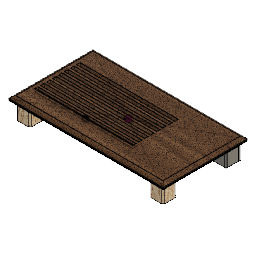
laotop-stand (Autodesk Fusion 360 design; units mm, degrees)
Autodesk Fusion 360 part; units mm, degrees
sketch "Sketch1" plane through (0, 0, 0) normal (0, 0, 1) x (1, 0, 0) in component "Top"
  line L0 (279.4, 152.4) -> (-279.4, 152.4)
  line L1 (-279.4, 152.4) -> (-279.4, -152.4)
  line L2 (-279.4, -152.4) -> (279.4, -152.4)
  line L3 (279.4, -152.4) -> (279.4, 152.4)
  line L4 (279.4, 152.4) -> (-279.4, -152.4) construction
  line L5 (-279.4, 152.4) -> (279.4, -152.4) construction
  line L6 (101.6, -84.6667) -> (-254, -84.6667)
  line L7 (-254, -84.6667) -> (-254, -71.9667)
  line L8 (-254, -71.9667) -> (101.6, -71.9667)
  line L9 (101.6, -71.9667) -> (101.6, -84.6667)
  line L10 (101.6, -84.6667) -> (-254, -71.9667) construction
  line L11 (-254, -84.6667) -> (101.6, -71.9667) construction
  point P0 (-76.2, -78.3167)
  dimension "d17" = 558.8
  dimension "d18" = 304.8
  dimension "d19" = 67.7333
  dimension "d20" = 25.4
  dimension "d21" = 355.6
  dimension "d22" = 12.7
  constraint perpendicular L0 L1
  constraint parallel L0 L2
  constraint parallel L1 L3
  constraint horizontal L0
  constraint coincident L4 origin
  constraint coincident L5 origin
  constraint perpendicular L6 L7
  constraint parallel L6 L8
  constraint parallel L7 L9
  constraint horizontal L6
  constraint coincident L10 P0
  constraint coincident L11 P0
  measures "d17" distance of L1.end L2.end
  measures "d18" distance of L0.end L1.end
  measures "d19" distance of L2 L6
  measures "d20" distance of L1 L7
  measures "d21" distance of L6.start L6.end
  measures "d22" distance of L6.end L7.end
extrude "Extrude1" add sketch "Sketch1" along normal mid plane 19.05 makes body 1 in component "Top"
pattern_linear "R-Pattern1" count 1 spacing 0 along (1, 0, 0) count 8 spacing 21.7714 along (0, 1, 0) of 4 faces at (-16.9333, -71.9667, -3.175) (-135.4667, -84.6667, -3.175) (-254, -80.4333, -3.175) (101.6, -76.2, -3.175) on bodies 1 in component "Top"
sketch "Sketch1 (2)" plane through (0, 0, -9.525) normal (0, 0, -1) x (-1, 0, 0) in component "Leg 1"
  line L0 (254, -67.7333) -> (254, -80.4333)
  line L1 (254, -80.4333) -> (-101.6, -80.4333)
  line L2 (-101.6, -80.4333) -> (-101.6, -67.7333)
  line L3 (-101.6, -67.7333) -> (254, -67.7333)
  line L4 (254, -45.9619) -> (254, -58.6619)
  line L5 (254, -58.6619) -> (-101.6, -58.6619)
  line L6 (-101.6, -58.6619) -> (-101.6, -45.9619)
  line L7 (-101.6, -45.9619) -> (254, -45.9619)
  line L8 (254, -24.1905) -> (254, -36.8905)
  line L9 (254, -36.8905) -> (-101.6, -36.8905)
  line L10 (-101.6, -36.8905) -> (-101.6, -24.1905)
  line L11 (-101.6, -24.1905) -> (254, -24.1905)
  line L12 (254, -2.419) -> (254, -15.119)
  line L13 (254, -15.119) -> (-101.6, -15.119)
  line L14 (-101.6, -15.119) -> (-101.6, -2.419)
  line L15 (-101.6, -2.419) -> (254, -2.419)
  line L16 (254, 19.3524) -> (254, 6.6524)
  line L17 (254, 6.6524) -> (-101.6, 6.6524)
  line L18 (-101.6, 6.6524) -> (-101.6, 19.3524)
  line L19 (-101.6, 19.3524) -> (254, 19.3524)
  line L20 (254, 41.1238) -> (254, 28.4238)
  line L21 (254, 28.4238) -> (-101.6, 28.4238)
  line L22 (-101.6, 28.4238) -> (-101.6, 41.1238)
  line L23 (-101.6, 41.1238) -> (254, 41.1238)
  line L24 (254, 62.8952) -> (254, 50.1952)
  line L25 (254, 50.1952) -> (-101.6, 50.1952)
  line L26 (-101.6, 50.1952) -> (-101.6, 62.8952)
  line L27 (-101.6, 62.8952) -> (254, 62.8952)
  line L28 (254, 71.9667) -> (-101.6, 71.9667)
  line L29 (-101.6, 71.9667) -> (-101.6, 84.6667)
  line L30 (-101.6, 84.6667) -> (254, 84.6667)
  line L31 (254, 84.6667) -> (254, 71.9667)
  line L32 (-279.4, 152.4) -> (-279.4, -152.4)
  line L33 (-279.4, -152.4) -> (279.4, -152.4)
  line L34 (279.4, -152.4) -> (279.4, 152.4)
  line L35 (279.4, 152.4) -> (-279.4, 152.4)
  line L36 (-215.9, -139.7) -> (-266.7, -139.7)
  line L37 (-266.7, -139.7) -> (-266.7, -88.9)
  line L38 (-266.7, -88.9) -> (-215.9, -88.9)
  line L39 (-215.9, -88.9) -> (-215.9, -139.7)
  line L40 (-279.4, 152.4) -> (-279.4, -152.4)
  line L41 (-279.4, -152.4) -> (279.4, -152.4)
  line L42 (-222.25, -131.2333) -> (-260.35, -131.2333)
  line L43 (-260.35, -131.2333) -> (-260.35, -121.0733)
  line L44 (-260.35, -121.0733) -> (-222.25, -121.0733)
  line L45 (-222.25, -121.0733) -> (-222.25, -131.2333)
  line L46 (-279.4, 152.4) -> (-279.4, -152.4)
  line L47 (-266.7, -114.3) -> (-215.9, -114.3) construction
  line L48 (-260.35, -107.5267) -> (-222.25, -107.5267)
  line L49 (-260.35, -97.3667) -> (-260.35, -107.5267)
  line L50 (-222.25, -97.3667) -> (-260.35, -97.3667)
  line L51 (-222.25, -107.5267) -> (-222.25, -97.3667)
  line L52 (-279.4, 0) -> (279.4, 0) construction
  line L53 (-266.7, 88.9) -> (-215.9, 88.9)
  line L54 (-222.25, 97.3667) -> (-260.35, 97.3667)
  line L55 (-266.7, 114.3) -> (-215.9, 114.3) construction
  line L56 (-222.25, 131.2333) -> (-260.35, 131.2333)
  line L57 (-215.9, 139.7) -> (-266.7, 139.7)
  line L58 (-215.9, 88.9) -> (-215.9, 139.7)
  line L59 (-222.25, 121.0733) -> (-222.25, 131.2333)
  line L60 (-260.35, 97.3667) -> (-260.35, 107.5267)
  line L61 (-222.25, 107.5267) -> (-222.25, 97.3667)
  line L62 (-260.35, 121.0733) -> (-222.25, 121.0733)
  line L63 (-260.35, 107.5267) -> (-222.25, 107.5267)
  line L64 (-260.35, 131.2333) -> (-260.35, 121.0733)
  line L65 (-266.7, 139.7) -> (-266.7, 88.9)
  line L66 (0, -152.4) -> (0, 152.4) construction
  line L67 (266.7, -139.7) -> (266.7, -88.9)
  line L68 (222.25, -121.0733) -> (222.25, -131.2333)
  line L69 (222.25, -107.5267) -> (222.25, -97.3667)
  line L70 (222.25, -131.2333) -> (260.35, -131.2333)
  line L71 (222.25, -97.3667) -> (260.35, -97.3667)
  line L72 (266.7, -88.9) -> (215.9, -88.9)
  line L73 (260.35, -107.5267) -> (222.25, -107.5267)
  line L74 (215.9, -139.7) -> (266.7, -139.7)
  line L75 (260.35, -121.0733) -> (222.25, -121.0733)
  line L76 (260.35, -131.2333) -> (260.35, -121.0733)
  line L77 (260.35, -97.3667) -> (260.35, -107.5267)
  line L78 (215.9, -88.9) -> (215.9, -139.7)
  line L79 (266.7, -114.3) -> (215.9, -114.3) construction
  line L80 (260.35, 107.5267) -> (222.25, 107.5267)
  line L81 (222.25, 131.2333) -> (260.35, 131.2333)
  line L82 (260.35, 131.2333) -> (260.35, 121.0733)
  line L83 (222.25, 121.0733) -> (222.25, 131.2333)
  line L84 (260.35, 97.3667) -> (260.35, 107.5267)
  line L85 (222.25, 97.3667) -> (260.35, 97.3667)
  line L86 (266.7, 139.7) -> (266.7, 88.9)
  line L87 (215.9, 139.7) -> (266.7, 139.7)
  line L88 (215.9, 88.9) -> (215.9, 139.7)
  line L89 (260.35, 121.0733) -> (222.25, 121.0733)
  line L90 (266.7, 88.9) -> (215.9, 88.9)
  line L91 (222.25, 107.5267) -> (222.25, 97.3667)
  line L92 (266.7, 114.3) -> (215.9, 114.3) construction
  line L93 (254, 80.4333) -> (254, 67.7333)
  line L94 (254, 67.7333) -> (-101.6, 67.7333)
  line L95 (-101.6, 67.7333) -> (-101.6, 80.4333)
  line L96 (-101.6, 80.4333) -> (254, 80.4333)
  line L97 (254, 58.6619) -> (254, 45.9619)
  line L98 (254, 45.9619) -> (-101.6, 45.9619)
  line L99 (-101.6, 45.9619) -> (-101.6, 58.6619)
  line L100 (-101.6, 58.6619) -> (254, 58.6619)
  line L101 (254, 36.8905) -> (254, 24.1905)
  line L102 (254, 24.1905) -> (-101.6, 24.1905)
  line L103 (-101.6, 24.1905) -> (-101.6, 36.8905)
  line L104 (-101.6, 36.8905) -> (254, 36.8905)
  line L105 (254, 15.119) -> (254, 2.419)
  line L106 (254, 2.419) -> (-101.6, 2.419)
  line L107 (-101.6, 2.419) -> (-101.6, 15.119)
  line L108 (-101.6, 15.119) -> (254, 15.119)
  line L109 (254, -6.6524) -> (254, -19.3524)
  line L110 (254, -19.3524) -> (-101.6, -19.3524)
  line L111 (-101.6, -19.3524) -> (-101.6, -6.6524)
  line L112 (-101.6, -6.6524) -> (254, -6.6524)
  line L113 (254, -28.4238) -> (254, -41.1238)
  line L114 (254, -41.1238) -> (-101.6, -41.1238)
  line L115 (-101.6, -41.1238) -> (-101.6, -28.4238)
  line L116 (-101.6, -28.4238) -> (254, -28.4238)
  line L117 (254, -50.1952) -> (254, -62.8952)
  line L118 (254, -62.8952) -> (-101.6, -62.8952)
  line L119 (-101.6, -62.8952) -> (-101.6, -50.1952)
  line L120 (-101.6, -50.1952) -> (254, -50.1952)
  line L121 (-101.6, -71.9667) -> (254, -71.9667)
  line L122 (254, -71.9667) -> (254, -84.6667)
  line L123 (254, -84.6667) -> (-101.6, -84.6667)
  line L124 (-101.6, -84.6667) -> (-101.6, -71.9667)
  line L125 (-279.4, 152.4) -> (-279.4, -152.4)
  line L126 (-279.4, -152.4) -> (279.4, -152.4)
  line L127 (279.4, -152.4) -> (279.4, 152.4)
  line L128 (279.4, 152.4) -> (-279.4, 152.4)
  dimension "d31" = 50.8
  dimension "d32" = 50.8
  dimension "d33" = 12.7
  dimension "d34" = 12.7
  dimension "d36" = 10.16
  dimension "d39" = 8.4667
  dimension "d40" = 6.35
  dimension "d41" = 6.35
  constraint horizontal L36
  constraint vertical L37
  constraint horizontal L38
  constraint vertical L39
  constraint horizontal L42
  constraint vertical L43
  constraint horizontal L44
  constraint vertical L45
  constraint midpoint L37 L47.start
  constraint midpoint L39 L47.end
  constraint symmetric L42.start L47 L50.start
  constraint symmetric L42.end L47 L49.start
  constraint symmetric L43.end L47 L48.start
  constraint symmetric L44.end L47 L48.end
  constraint midpoint L32 L52.start
  constraint midpoint L34 L52.end
  constraint symmetric L36.start L52 L57.start
  constraint symmetric L36.end L52 L57.end
  constraint symmetric L37.end L52 L53.start
  constraint symmetric L38.end L52 L53.end
  constraint symmetric L42.start L52 L56.start
  constraint symmetric L42.end L52 L56.end
  constraint symmetric L43.end L52 L62.start
  constraint symmetric L44.end L52 L59.start
  constraint symmetric L47.start L52 L55.start
  constraint symmetric L47.end L52 L55.end
  constraint symmetric L48.start L52 L60.end
  constraint symmetric L48.end L52 L61.start
  constraint symmetric L49.start L52 L54.end
  constraint symmetric L50.start L52 L54.start
  constraint midpoint L41 L66.start
  constraint midpoint L35 L66.end
  constraint symmetric L36.start L66 L74.start
  constraint symmetric L36.end L66 L67.start
  constraint symmetric L37.end L66 L67.end
  constraint symmetric L38.end L66 L72.end
  constraint symmetric L42.start L66 L68.end
  constraint symmetric L42.end L66 L70.end
  constraint symmetric L43.end L66 L75.start
  constraint symmetric L44.end L66 L68.start
  constraint symmetric L47.start L66 L79.start
  constraint symmetric L47.end L66 L79.end
  constraint symmetric L48.start L66 L73.start
  constraint symmetric L48.end L66 L69.start
  constraint symmetric L49.start L66 L71.end
  constraint symmetric L50.start L66 L69.end
  constraint symmetric L62.start L66 L82.end
  constraint symmetric L57.end L66 L86.start
  constraint symmetric L53.start L66 L86.end
  constraint symmetric L56.end L66 L81.end
  constraint symmetric L56.start L66 L81.start
  constraint symmetric L53.end L66 L88.start
  constraint symmetric L54.start L66 L85.start
  constraint symmetric L54.end L66 L84.start
  constraint symmetric L61.start L66 L80.end
  constraint symmetric L60.end L66 L80.start
  constraint symmetric L55.end L66 L92.end
  constraint symmetric L55.start L66 L92.start
  constraint symmetric L57.start L66 L87.start
  constraint symmetric L59.start L66 L83.start
  measures "d31" distance of L36.start L36.end
  measures "d32" distance of L36.start L38.end
  measures "d33" distance of L37 L40
  measures "d34" distance of L36 L41
  measures "d36" distance of L42.start L44.end
  measures "d39" distance of L36 L42
  measures "d40" distance of L37 L43
  measures "d41" distance of L39 L45
extrude "Extrude1'" add sketch "Sketch1 (2)" along normal blind 57.15 separate body contours L53 L57 L58 L65 | L54 L60 L61 L63 | L56 L59 L62 L64 makes body 2 in component "Leg 1"
extrude "Extrude2" add sketch "Sketch1 (2)" against normal blind 12.7 separate body contours L54 L60 L61 L63 | L56 L59 L62 L64 makes body 3 at (247.65, 121.0733, -5.2917) makes body 4 at (234.95, 97.3667, -5.2917) in component "Leg 1"
combine "Combine1" operation add target body 3 tool bodies 4 2 keep tools in component "Leg 1"
combine "Combine2" operation add target body 4 tool bodies 2 3 keep tools in component "Leg 1"
combine "Combine1'" operation add target body 1 tool bodies 3 keep tools in component "Top"
combine "Combine2'" operation cut target body 1 tool bodies 4 keep tools in component "Top"
extrude "Extrude3" add sketch "Sketch1 (2)" along normal blind 57.15 separate body contours L36 L37 L38 L39 | L42 L43 L44 L45 | L48 L49 L50 L51 makes body 5 in component "Leg 1"
extrude "Extrude4" add sketch "Sketch1 (2)" against normal blind 12.7 contours L42 L43 L44 L45 | L48 L49 L50 L51 bodies 5 in component "Leg 1"
combine "Combine3" operation cut target body 1 tool bodies 5 keep tools in component "Top"
extrude "Extrude5" add sketch "Sketch1 (2)" along normal blind 57.15 separate body contours L67 L72 L74 L78 | L68 L70 L75 L76 | L69 L71 L73 L77 makes body 6 in component "Leg 1"
extrude "Extrude6" add sketch "Sketch1 (2)" against normal blind 12.7 contours L68 L70 L75 L76 | L69 L71 L73 L77 bodies 6 in component "Leg 1"
combine "Combine4" operation cut target body 1 tool bodies 6 keep tools in component "Top"
extrude "Extrude7" add sketch "Sketch1 (2)" along normal blind 57.15 separate body contours L80 L84 L85 L91 | L81 L82 L83 L89 | L86 L87 L88 L90 makes body 7 in component "Leg 1"
extrude "Extrude8" add sketch "Sketch1 (2)" against normal blind 12.7 contours L80 L84 L85 L91 | L81 L82 L83 L89 bodies 7 in component "Leg 1"
combine "Combine5" operation cut target body 1 tool bodies 7 keep tools in component "Top"
fillet "Fillet1" radius 12.7 4 edges at (0, 152.4, 9.525) (-279.4, 0, 9.525) (0, -152.4, 9.525) (279.4, 0, 9.525) on bodies 1 in component "Top"
chamfer "Chamfer1" distance 6.35 angle 45 16 edges at (266.7, 139.7, -38.1) (266.7, 88.9, -38.1) (215.9, 139.7, -38.1) (215.9, 88.9, -38.1) (-215.9, -139.7, -38.1) (-215.9, -88.9, -38.1) (-266.7, -139.7, -38.1) (-266.7, -88.9, -38.1) (215.9, -88.9, -38.1) (215.9, -139.7, -38.1) (266.7, -139.7, -38.1) (266.7, -88.9, -38.1) (-215.9, 88.9, -38.1) (-215.9, 139.7, -38.1) (-266.7, 88.9, -38.1) (-266.7, 139.7, -38.1) on bodies 4 5 6 7 in component "Leg 1"
chamfer "Chamfer1'" distance 3.175 angle 45 4 edges at (279.4, 0, -9.525) (0, -152.4, -9.525) (0, 152.4, -9.525) (-279.4, 0, -9.525) on bodies 1 in component "Top"
component "Top" placed x (1, 0, 0) y (0, 1, 0) z (0, 0, 1) at (0, 0, 0)
component "Leg 1" placed x (1, 0, 0) y (0, 1, 0) z (0, 0, 1) at (0, 0, 0)
equation "TopWidth = 22 in"
equation "TopLength = 12 in"
equation "TopThickness = ( 3 / 4 ) * 1 in"
equation "OverallHeight = 3 in"
equation "SlotWidth = ( 1 / 2 ) * 1 in"
equation "SlotLength = 14 in"
equation "SlotOffsetFront = 2 in + ( 2 / 3 ) * 1 in"
equation "SlotOffsetSide = 1 in"
equation "SlotSpacing = 1 in"
equation "LegWidth = 2 in"
equation "LegOffset = ( 1 / 2 ) * 1 in"
equation "LegTenonLength = LegWidth * 2 / 3"
equation "LegTenonWidth = LegWidth / 5"
equation "LegTenonOffsetFront = ( 1 / 3 ) * 1 in"
equation "LegTenonOffsetSide = ( 1 / 4 ) * 1 in"
equation "LegTenonHeight = TopThickness * 2 / 3"
equation "d17 = TopWidth"
equation "d18 = TopLength"
equation "d19 = SlotOffsetFront"
equation "d20 = SlotOffsetSide"
equation "d21 = SlotLength"
equation "d22 = SlotWidth"
equation "d24 = TopThickness / 2"
equation "d27 = NumSlots"
equation "NumSlots = 8"
equation "d31 = LegWidth"
equation "d32 = LegWidth"
equation "d33 = LegOffset"
equation "d34 = LegOffset"
equation "d36 = LegTenonWidth"
equation "d39 = LegTenonOffsetFront"
equation "d40 = LegTenonOffsetSide"
equation "d41 = LegTenonOffsetSide"
equation "d42 = OverallHeight - TopThickness"
equation "d44 = -LegTenonHeight"
equation "d46 = OverallHeight - TopThickness"
equation "d48 = -LegTenonHeight"
equation "d50 = OverallHeight - TopThickness"
equation "d52 = -LegTenonHeight"
equation "d54 = OverallHeight - TopThickness"
equation "d56 = -LegTenonHeight"
